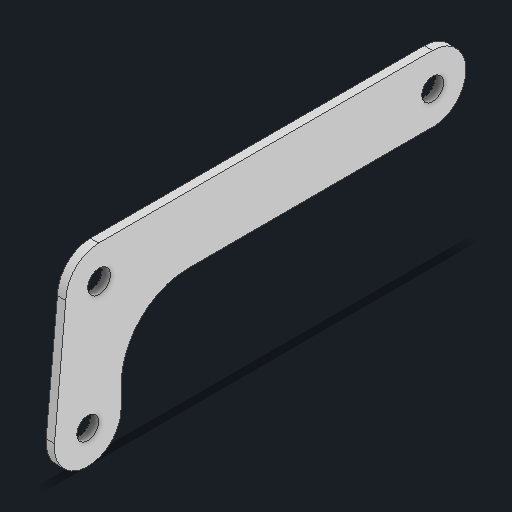
# Autodesk Inventor part: Passive Gusset
Saved by Autodesk Inventor 2025.1 (Build 291241000, 241)
## iProperties
Created: 2024-10-24
Part Number: Passive Gusset
Material: Generic
Document SubType Name: Modeling
Designer: avere
Density: 1 g/cm^3
Appearance: Default
d0: 0.500 in
d1: 0.500 in
d2: 0.500 in
d3: 0.165 in
d4: 0.165 in
Author: avere
Autodesk Inventor part; units mm, degrees
ref_plane "YZ Plane" through (0, 0, 0) normal (1, 0, 0) x (0, 1, 0)
ref_plane "XZ Plane" through (0, 0, 0) normal (0, 1, 0) x (-1, 0, 0)
ref_plane "XY Plane" through (0, 0, 0) normal (0, 0, 1) x (1, 0, 0)
sketch "main" plane through (0, 0, 0) normal (0, 0, 1) x (1, 0, 0)
  circle A0 centre (33.3179, -13.5957) radius 2.1844
  arc A1 (33.2126, -19.9448) -> (39.6679, -13.5957) centre (33.3179, -13.5957) ccw
  arc A2 (-29.1607, -7.2457) -> (-30.1903, -19.863) centre (-30.1821, -13.513) ccw
  arc A3 (41.8234, 8.9199) -> (29.1525, 9.5788) centre (35.5023, 9.525) ccw
  line L0 (39.6679, -13.5957) -> (41.8234, 8.9199)
  line L1 (-29.1607, -7.2457) -> (16.4171, -7.2457)
  line L2 (29.1166, 5.3466) -> (29.1525, 9.5788)
  arc A4 (16.4171, -7.2457) -> (29.1166, 5.3466) centre (16.4171, 5.4543) ccw
  circle A5 centre (35.5023, 9.525) radius 2.0955
  line L3 (33.4068, -19.9451) -> (-30.1903, -19.863)
  circle A6 centre (-30.1821, -13.513) radius 2.0955
  point P0 (20.4908, -8.19)
  dimension "d0" = 12.7
  dimension "d1" = 12.7
  dimension "d2" = 12.7
  dimension "d3" = 4.191
  dimension "d4" = 4.191
  measures "d0" diameter of A1
  measures "d1" diameter of A3
  measures "d2" radius of A4
  measures "d3" diameter of A5
  measures "d4" diameter of A6
sketch "Sketch1" plane through (0, 0, 0) normal (1, 0, 0) x (0, 1, 0)
  circle A0 centre (0.0357, 63.5) radius 2.1844
  arc A1 (6.3849, 63.3995) -> (0.031, 69.85) centre (0.0357, 63.5) ccw
  arc A2 (-6.2681, 1.0168) -> (6.35, -0.0035) centre (0, 0) ccw
  arc A3 (-22.4861, 71.9889) -> (-23.1357, 59.3175) centre (-23.0866, 65.6674) ccw
  line L0 (0.031, 69.85) -> (-22.4861, 71.9889)
  line L1 (-6.2681, 1.0168) -> (-6.3018, 46.5946)
  line L2 (-18.9035, 59.2848) -> (-23.1357, 59.3175)
  arc A4 (-6.3018, 46.5946) -> (-18.9035, 59.2848) centre (-19.0018, 46.5852) ccw
  circle A5 centre (-23.0866, 65.6674) radius 2.0955
  line L3 (6.385, 63.5936) -> (6.35, -0.0035)
  circle A6 centre (0, 0) radius 2.0955
  point P0 (0, 0)
  constraints: 1 other
extrude "Extrusion1" add sketch "Sketch1" along normal blind 1.5875
body "Solid1"
